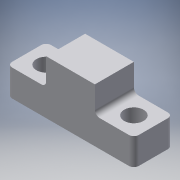
# Autodesk Inventor part: Left half
Saved by Autodesk Inventor 2018 (Build 220112000, 112)
## iProperties
Created: 2005-07-15
Part Number: Left half
Document SubType Name: Modeling
Designer: Administrator
Manufacturer: Standard
Standards Organization: Custom
Material: Generic
Density: 1 g/cm^3
Appearance: Cool White
Author: Administrator
Autodesk Inventor part; units mm, degrees
ref_plane "YZ Plane" through (0, 0, 0) normal (1, 0, 0) x (0, 1, 0)
ref_plane "XZ Plane" through (0, 0, 0) normal (0, 1, 0) x (-1, 0, 0)
ref_plane "XY Plane" through (0, 0, 0) normal (0, 0, 1) x (1, 0, 0)
sketch "Sketch1" plane through (0, 0, 0) normal (0, 0, 1) x (1, 0, 0)
  line L0 (0, -14.2875) -> (0, 20.6375)
  line L1 (0, 20.6375) -> (-15.875, 20.6375)
  line L2 (-15.875, 20.6375) -> (-15.875, 3.175)
  line L3 (-15.875, 3.175) -> (-41.275, 3.175)
  line L4 (-41.275, 3.175) -> (-41.275, -14.2875)
  line L5 (-41.275, -14.2875) -> (0, -14.2875)
  constraints: 12 end point, 4 parallel, 1 perpendicular, 1 vertical
extrude "Extrusion1" add sketch "Sketch1" along normal blind 25.4
sketch "Sketch2" plane through (-41.275, 3.175, 0) normal (0, 1, 0) x (1, 0, 0)
  circle A0 centre (12.7, -12.7) radius 6.35
  constraints: 1 centre point
extrude "Extrusion2" cut sketch "Sketch2" against normal through all
fillet "Fillet1" radius 3.175 3 edges at (-41.275, -5.5563, 25.4) (-41.275, -5.5563, 0) (-15.875, 3.175, 12.7)
mirror "Mirror1" about plane through (0, 20.6375, 0) normal (1, 0, 0) of "Extrusion1", "Extrusion2", "Fillet1"
body "Solid1"
